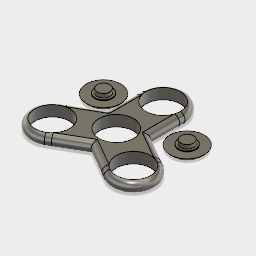
FidgetSpinnerV1 v1 (Autodesk Fusion 360 design; units mm, degrees)
Autodesk Fusion 360 part; units mm, degrees
sketch "Sketch1" plane through (0, 0, 0) normal (0, 1, 0) x (1, 0, 0)
  line L0 (-13.8843, 14.8996) -> (14.1157, 14.8996)
  line L1 (14.1157, 14.8996) -> (14.1157, -15.1004)
  line L2 (14.1157, -15.1004) -> (-13.8843, -15.1004)
  line L3 (-13.8843, -15.1004) -> (-13.8843, 14.8996)
  circle A0 centre (0.1157, 14.8996) radius 14
  circle A1 centre (0.1157, 14.8996) radius 11.025
  circle A2 centre (0.1157, -15.1004) radius 14
  circle A3 centre (0.1157, -15.1004) radius 11.025
  dimension "d1" = 28
  dimension "d2" = 30
  dimension "d3" = 28
  dimension "d4" = 22.05
  dimension "d5" = 28
  dimension "d6" = 22.05
  measures "d1" distance of L0.start L0.end
  measures "d2" distance of L0.start L2.end
  measures "d3" diameter of A0
  measures "d4" diameter of A1
  measures "d5" diameter of A2
  measures "d6" diameter of A3
extrude "Extrude1" add sketch "Sketch1" along normal blind 7 contours L0 A0 A1 | L0 A0 A1 | L1 L3 A0 A2 | L2 A2 A3 | L2 A2 A3 makes body 1
pattern_circular "C-Pattern1" count 3 over 360 about axis through (0.1157, 0, 15.1004) along (0, 1, 0) of bodies 1 makes body 2 at (-16.2476, 0, 9.9473) makes body 3 at (22.3775, 0, 13.3527)
combine "Combine1" operation add target body 1 tool bodies 2 3
sketch "Sketch2" plane through (0, 0, 0) normal (0, 1, 0) x (1, 0, 0)
  circle A0 centre (-27.7152, 4.586) radius 11
  circle A1 centre (-27.7152, 4.586) radius 5.5
  circle A2 centre (-27.7152, 4.586) radius 4.075
  dimension "d11" = 22
  dimension "d12" = 11
  dimension "d13" = 8.15
  measures "d11" diameter of A0
  measures "d12" diameter of A1
  measures "d13" diameter of A2
extrude "Extrude2" add sketch "Sketch2" along normal blind 2.5 separate body contours A0 makes body 4
extrude "Extrude3" add sketch "Sketch2" along normal blind 3 contours A1 bodies 4
extrude "Extrude4" add sketch "Sketch2" along normal blind 5.5 contours A2 bodies 4
fillet "Fillet1" radius 3.5 18 edges at (-9.3747, 0, 36.7454) (-37.9894, 0, 37.1004) (-23.3747, 0, 12.4967) (-23.3747, 7, 12.4967) (-37.9894, 7, 37.1004) (-9.3747, 7, 36.7454) (9.6061, 7, 36.7454) (38.2208, 7, 37.1004) (23.6061, 7, 12.4967) (23.6061, 0, 12.4967) (38.2208, 0, 37.1004) (9.6061, 0, 36.7454) (14.1157, 7, -3.9411) (0.1157, 7, -28.8996) (-13.8843, 7, -3.9411) (-13.8843, 0, -3.9411) (0.1157, 0, -28.8996) (14.1157, 0, -3.9411) on bodies 1
fillet "Fillet2" radius 3.5 1 edges at (-37.9708, 0, -0.6082) on bodies 4
extrude "Extrude5" cut 1 faces at (-29.7077, 0, -5.2704) along direction (0, 1, 0) blind 0.5 on bodies 4 bodies 4
fillet "Fillet3" radius 1 1 edges at (-20.5867, 0, -7.3508) on bodies 4
fillet "Fillet4" radius 1 1 edges at (-20.5867, 0.5, -7.3508) on bodies 4
copy_body "CopyPasteBodies1" bodies 4 makes body 5
move_body "Move1" bodies 5 to x (1, 0, 0) y (0, 1, 0) z (0, 0, 1) at (55.0932, 0, 1.5741)
